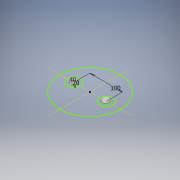
# Autodesk Inventor part: Eyes
Saved by Autodesk Inventor 2018.2 (Build 222227000, 227)
## iProperties
Created: 2018-02-13
Part Number: Eyes
Material: Generisch
Document SubType Name: Modeling
Designer: JochenAlt
Density: 1 g/cm^3
Appearance: Vorgabe
Author: JochenAlt
Autodesk Inventor part; units mm, degrees
ref_plane "YZ Plane" through (0, 0, 0) normal (1, 0, 0) x (0, 1, 0)
ref_plane "XZ Plane" through (0, 0, 0) normal (0, 1, 0) x (-1, 0, 0)
ref_plane "XY Plane" through (0, 0, 0) normal (0, 0, 1) x (1, 0, 0)
sketch "Skizze1" plane through (0, 0, 0) normal (0, 0, 1) x (1, 0, 0)
  circle A0 centre (-50, 0) radius 10
  line L0 (0, 128.4817) -> (0, -128.4817) construction
  circle A1 centre (50, 0) radius 10
  line L1 (-60, 0) -> (-40, 0)
  line L2 (40, 0) -> (60, 0)
  line L3 (-128.4817, 0) -> (128.4817, 0) construction
  circle A2 centre (-50, 0) radius 20
  circle A3 centre (50, 0) radius 20
  circle A4 centre (0, 0) radius 91.7726
  dimension "d0" = 20
  dimension "d1" = 100
  dimension "d3" = 40
  constraints: 5 centre point, 4 end point, 4 point on circle, 3 coincident, 2 equal radius, 2 horizontal, 1 midpoint, 1 other
  measures "d0" diameter of A0
  measures "d1" distance of A1.centre A0.centre
  measures "d3" diameter of A2
revolve "Umdrehung1" add sketch "Skizze1" angle 180 about axis through (0, 0, 0) along (1, 0, 0) picked at (-52.6218, 5.86) picked at (47.3782, 5.86) contours L1 A0 | L2 A1
extrude "Extrusion1" cut sketch "Skizze1" against normal blind 1 contours L1 A0 | A0 L1 | L2 A1 | A1 L2 | A2 | A3
extrude "Extrusion2" cut sketch "Skizze1" along normal blind 1 contours L1 A0 | A0 L1 | L2 A1 | A1 L2 | A2 | A3
extrude "Extrusion3" add sketch "Skizze1" against normal blind 5 contours A4
